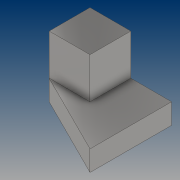
# Autodesk Inventor part: 3
Saved by Autodesk Inventor 2020.2 (Build 242310000, 310)
## iProperties
Created: 2020-09-17
Part Number: 3
Material: 鋼、碳鋼
Document SubType Name: Modeling
Designer: user
Density: 7.85 g/cm^3
Appearance: 半拋光
Mass: 157 g
Surface Area: 54.4721 cm^2
Volume: 20 cm^3
Author: user
Autodesk Inventor part; units mm, degrees
ref_plane "YZ Plane" through (0, 0, 0) normal (1, 0, 0) x (0, 1, 0)
ref_plane "XZ Plane" through (0, 0, 0) normal (0, 1, 0) x (-1, 0, 0)
ref_plane "XY Plane" through (0, 0, 0) normal (0, 0, 1) x (1, 0, 0)
sketch "草圖1" plane through (0, 0, 0) normal (0, 1, 0) x (-1, 0, 0)
  line L0 (-20, 20) -> (20, 20)
  line L1 (20, 20) -> (20, -20)
  line L2 (20, -20) -> (-20, -20)
  line L3 (-20, -20) -> (-20, 20)
  line L4 (-20, 20) -> (20, -20) construction
  line L5 (20, 20) -> (-20, -20) construction
  point P0 (0, 0)
  dimension "d0" = 40
  dimension "d1" = 40
  constraints: 12 end point, 2 midpoint, 2 parallel, 1 horizontal, 1 perpendicular
  measures "d0" distance of L0.start L0.end
  measures "d1" distance of L2.end L0.start
extrude "擠出1" add sketch "草圖1" along normal blind 10
sketch "草圖2" plane through (0, 10, 0) normal (0, 1, 0) x (1, 0, 0)
  line L0 (-20, 20) -> (20, 20) projected
  line L1 (20, 20) -> (20, -20) projected
  line L2 (20, -20) -> (-20, -20) projected
  line L3 (-20, -20) -> (-20, 20) projected
  line L4 (20, 20) -> (-20, 20) projected
  line L5 (-20, 20) -> (0, 20)
  line L6 (0, 20) -> (0, 0)
  line L7 (0, 0) -> (-20, 0)
  line L8 (-20, 0) -> (-20, 20)
  point P0 (0, 0)
  point P1 (0, 20)
  dimension "d4" = 20
  dimension "d5" = 20
  constraints: 8 end point, 2 parallel, 1 horizontal, 1 perpendicular
  measures "d4" distance of L6.end L7.end
  measures "d5" distance of L5.end L6.end
extrude "擠出2" add sketch "草圖2" along normal blind 20 contours L0 L6 L7 L3
sketch "草圖3" plane through (0, 10, 0) normal (0, 1, 0) x (1, 0, 0)
  line L0 (0, 20) -> (0, 0) projected
  line L1 (0, 0) -> (-20, 0) projected
  line L2 (-20, -20) -> (-20, 0) projected
  line L3 (20, -20) -> (-20, -20) projected
  line L4 (20, 20) -> (20, -20) projected
  line L5 (0, 20) -> (20, 20) projected
  line L6 (-20, 20) -> (0, 20) projected
  line L7 (-20, 0) -> (-20, 20) projected
  line L8 (20, -20) -> (20, 20) projected
  line L9 (-20, 0) -> (20, -20)
  constraints: 2 end point
extrude "擠出3" cut sketch "草圖3" against normal through all contours L9 L3 L2
